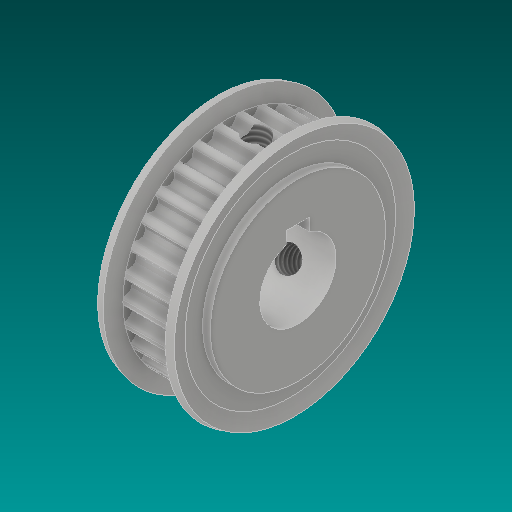
# Autodesk Inventor part: HTPA30S3M060-A-N10_b
Saved by Autodesk Inventor 2020 (Build 240168000, 168)
## iProperties
Created: 2022-11-15
Part Number: HTPA30S3M060-A-N10_b
Material: Generic
Catalog Web Link: www.cadenas.de
Description: HTPA__S3M060, HTPA__S3M100, HTPA__S3M150, HTPB__S3M060, HTPB__S3M100, HTPB__S3M150, HTPK__S3M060, HTPK__S3M100, HTPK__S3M150, HTPN__S3M060, HTPN__S3M100, HTPN__S3M150, HTPT__S3M060, HTPT__S3M100, HTPT__S3M150, HTPM__S3M060, HTPM__S3M100, HTPM__S3M150, HTPP__S3M060, HTPP__S3M100, HTPP__S3M150, HTPS__S3M060, HTPS__S3M100, KHTPA__S3M060, KHTPA__S3M100, KHTPA__S3M150, KHTPK__S3M060, KHTPK__S3M100, KHTPK__S3M150_body-High Torque Timing Pulleys S3M Type
Vendor: MISUMI
Document SubType Name: Modeling
Designer: psAdmin
Manufacturer: MISUMI
Mass: 5.31734 g
Surface Area: 36.0109 cm^2
Volume: 5.31734 cm^3
Density: 1 g/cm^3
Appearance: PSOLRGB-175-175-175
Category: PARTsolutions
Company: MISUMI
PSOL_IDENT_0: {$CADENAS_DATA/23d-libs/misumi/metric/51_timing_pulleys/htpk_s3m/htpa_s3m.prj},837 {VTYP=3D},{NB=HTP
PSOL_IDENT_1: A30S3M060-A-N10_b},{LINA=HTPA30S3M060-A-N10},{NN=HTPA__S3M060, HTPA__S3M100, HTPA__S3M150, HTPB__S3M
PSOL_IDENT_2: 060, HTPB__S3M100, HTPB__S3M150, HTPK__S3M060, HTPK__S3M100, HTPK__S3M150, HTPN__S3M060, HTPN__S3M10
PSOL_IDENT_3: 0, HTPN__S3M150, HTPT__S3M060, HTPT__S3M100, HTPT__S3M150, HTPM__S3M060, HTPM__S3M100, HTPM__S3M150,
PSOL_IDENT_4: HTPP__S3M060, HTPP__S3M100, HTPP__S3M150, HTPS__S3M060, HTPS__S3M100, KHTPA__S3M060, KHTPA__S3M100,
PSOL_IDENT_5: KHTPA__S3M150, KHTPK__S3M060, KHTPK__S3M100, KHTPK__S3M150_body},{DATE=28.10.2022 00:10:57},{GEOMDA
PSOL_IDENT_6: TE=11.11.2021 09:52:43},{VERSION=},{LINEID=160},{WBVAR=MATP,ST,TNW,PS,SBS,DD,Z,J,Q,R,S,T,ALT1,ALT2,M
PSOL_IDENT_7: ,QSC,QFC,QTC,ALT3,K,KSC,KFC,KTC,ALT4,ZM,ZSC,ZFC,ZTC,ALT5,ALT6,ALT7,FC,ALT8,SRG,ALT9,BTC,TL,ALT10,TPC
PSOL_IDENT_8: ,ALT11,BC,ALT12,SLH,ALT13,BN},{WBNUMERIC=DD,Z,J,Q,R,S,T,QSC,QFC,QTC,K,KSC,KFC,KTC,ZSC,ZFC,ZTC,FC,SRG
PSOL_IDENT_9: ,BTC,TL,BC,SLH,BN}  {NB=HTPA30S3M060-A-N10_b},{LINA=HTPA30S3M060-A-N10},{KT=DUMMY},{PN=HTPA30S3M060-
PSOL_IDENT_10: A-N10},{TYPE=HTPA},{MATP=A2017},{MATPALG='A2017','Aluminum Alloy 2000 series','S45C','1045 Carbon St
PSOL_IDENT_11: eel Equivalent','SUS304','304 Stainless Steel','A6000','6000 Series Aluminum Alloy'},{ST=CA},{STALG=
PSOL_IDENT_12: 'CA','Clear Anodize','BA','Black Anodize','HAT','Hard Clear Anodize','ENP','Electroless Nickel Plat
PSOL_IDENT_13: ing' },{NT=30},{TNW=S3M060},{TNWALG= 'S3M060','S3M100','S3M150'    },{BW=6},{PS=A},{PSALG='A','B'},{
PSOL_IDENT_14: SBS=N},{SBSALG= 'H','Round Hole','P','Round Hole + Tap','N','New JIS Keywayed Bore + Tap (Standard)'
PSOL_IDENT_15: ,'NK','New JIS Keywayed Bore + Tap (width 4.0mm, height 1.8mm)','C','Old JIS Keywayed Bore + Tap','V'
PSOL_IDENT_16: ,'Stepped Hole', 'Y','Both Ends Stepped Hole','WB', 'Double Stepped Hole' },{SHSA= 'H','Round Hole','
PSOL_IDENT_17: P','Round Hole + Tap','N','New JIS Keywayed Bore + Tap (Standard)','NK','New JIS Keywayed Bore + Tap
PSOL_IDENT_18: (width 4.0mm, height 1.8mm)','C','Old JIS Keywayed Bore + Tap','V','Stepped Hole', 'Y','Both Ends S
PSOL_IDENT_19: tepped Hole','WB', 'Double Stepped Hole' },{SHSB= 'H','Round Hole','P','Round Hole + Tap','N','New J
PSOL_IDENT_20: IS Keywayed Bore + Tap (Standard)','NK','New JIS Keywayed Bore + Tap (width 4.0mm, height 1.8mm)','C'
PSOL_IDENT_21: ,'Old JIS Keywayed Bore + Tap','V','Stepped Hole', 'F','Stepped Hole (Counterbore holes on the boss
PSOL_IDENT_22: side)'},{SHSK= '','' },{SBSPN=-N10},{DD=10.00},{DDALG=[8:8/1],[10:14/1]},{DDHA=[6:6/1],6.35,[7:12/1]
PSOL_IDENT_23: ,12.7,[13:19/1]},{DDHBK=0},{DDPA=[6:6/1],6.35,[7:12/1],12.7,[13:19/1]},{DDPBK=0},{DDNA=[8:8/1],[10:1
PSOL_IDENT_24: 4/1]},{DDNBK=0},{DDNK=10},{DDCA=[10:10/1],[12:12/1]},{DDCBK=0},{DDVA=[6:6/1],6.35,[7:12/1],12.7,[13:
PSOL_IDENT_25: 17/1]},{DDVF=[6:6/1],6.35,[7:12/1],12.7,[13:14/1]},{DDY=[6:17/1]},{DDWB=[6:15/1]},{Z=0},{ZALG=[0]},{
PSOL_IDENT_26: ZQRMIN=12},{ZAMAX=19},{ZBMAX=16},{DDZ=10},{J=0.0},{JALG=[0]},{JMAX=9},{JMIN=2},{JPN=},{QRMAX=19},{QR
PSOL_IDENT_27: MIN=12},{WBRMAX=-2.00},{WBQMIN=14},{Q=0},{QALG=[0]},{QPN=},{R=0},{RALG=[0]},{S=0.0},{SALG=[0]},{SPN=
PSOL_IDENT_28: },{SMAX=5},{T=0.0},{TALG=[0]},{TPN=},{TMAX=8},{A=7},{W=11},{L=0},{PD=28.65},{OD=27.89},{D=0},{DALG=2
PSOL_IDENT_29: 0},{DE=23},{F=32},{E=23},{BBK=3.000},{TTK=1.4},{TT=1},{ANG=120},{WL=11},{ALT1=},{ALT1ALG= '','w/o KC
PSOL_IDENT_30: 90 (Set Screw Angle)','KC90','with KC90 (Set Screw Angle)' },{ALT1PN=},{ALT2=},{ALT2ALG= '','Not app
PSOL_IDENT_31: licable' },{M=N/A},{MALG= 'N/A' },{MFTALG= 'N/A' },{MSALG= 'N/A' },{M3D=0.000},{KDML=0},{ML=0},{MUL=
PSOL_IDENT_32: 0},{PITCH=0},{QSC=0.0},{QSCALG=0},{QFC=0.0},{QFCALG=0},{QTC=0.0},{QTCALG=0},{QPCDMIN=0},{QPCDMINALG=
PSOL_IDENT_33: 0},{QPCDMAX=19},{ALT2PN=},{ALT3=},{ALT3ALG= '','Not applicable' },{K=0.0},{KALG=0},{KMIN=4},{KFTMAX=
PSOL_IDENT_34: 0.0},{KSMAX=0.0},{KSC=0.0},{KSCALG=0},{KFC=0.0},{KFCALG=0},{KTC=0.0},{KTCALG=0},{KPCDMIN=14},{KPCDMI
PSOL_IDENT_35: NALG=14},{KPCDMAX=19},{KSCMIN=14.0},{KSCMINALG=14},{ALT3PN=},{ALT4=},{ALT4ALG= '','Not applicable' }
PSOL_IDENT_36: ,{ALT4MIN=20.5},{ALT4MAX=12.5},{ZM=N/A},{ZMALG= 'N/A' },{ZMSALG= 'N/A' },{ZMFTALG= 'N/A' },{ZMDD1=0.
PSOL_IDENT_37: 0},{ZMDD2=0.0},{ZMHH=0.0},{ZSC=0.0},{ZSCALG=[0]},{ZFC=0.0},{ZFCALG=[0]},{ZTC=0.0},{ZTCALG=[0]},{ZPCD
PSOL_IDENT_38: MIN=0},{ZPCDMINALG=0},{ZPCDMAX=19},{ALT4PN=},{ALT5=},{ALT5ALG= '','Flange Attached','NFC','with NFC
PSOL_IDENT_39: (Flange not Attached)' },{ALT5PN=},{ALT6=},{ALT6ALG= '','w/o Flange Attached on One Side Only','RFC'
PSOL_IDENT_40: ,'with RFC (Flange Attached on The Boss Side Only)','LFC','with LFC (Flange Attached on The Opposite
PSOL_IDENT_41: Side Only)' },{ALT6PN=},{ALT7=},{ALT7ALG= '','w/o FC (Flange Cut)','FC','with FC (Flange Cut)' },{F
PSOL_IDENT_42: C=0.0},{FCALG=0},{FCMIN=29.0},{FCMAX=30.0},{ALT7PN=},{ALT8=},{ALT8ALG= '','Not applicable' },{ALT8AL
PSOL_IDENT_43: GALG=19},{ALT8DD2=0},{ALT8MM=0},{ALT8NN=0},{QC=0},{KC=0},{ZC=0},{SRG=0.0},{SRGALG=[0]},{SRGMAX1=0},{
PSOL_IDENT_44: SRGMAX=0},{DD2=0.0},{MM=0.00},{NN=0.00},{ALT8PN=},{ALT9ALG= '','Not applicable' },{ALT9=},{BTC9=11},
PSOL_IDENT_45: {TL9=1},{BTC=0},{BTCALG=[0]},{TL=0.0},{TLALG=0},{TLMIN=1.0},{TLMAX=-11.5},{BTCL=0},{BTCD=0},{BTCDALG=
PSOL_IDENT_46: 20.000},{ALT9PN=},{WLBCTL=11},{ALT10=},{ALT10ALG= '','w/o TPC (Tapped Hole Dimension)','TPC','with T
PSOL_IDENT_47: PC (Tapped Hole Dimension)' },{TPC=N/A},{TPCALG= 'N/A' },{TPCM=4},{ALT10PN=},{ALT11=},{ALT11ALG= '','
PSOL_IDENT_48: Not applicable' },{BC=0.0},{BCALG=0},{BCMIN=7},{BCMAX=-11.5},{BCPLANE=5.5},{M1WBC=5.5},{ALT11PN=},{A
PSOL_IDENT_49: LT12=},{ALT12ALG= '','w/o SLH (Set Screw Length)','SLH','with SLH (Set Screw Length)' },{SLH=0},{SLH
PSOL_IDENT_50: ALG=[0]},{ALT12PN=},{AC=M4x3},{M1=4},{M1L=3},{TAP=0.000},{KYY=5},{KTT=8.945},{PLANE=11},{CD=0},{ALT1
PSOL_IDENT_51: 3=},{ALT13ALG= '', 'Not applicable' },{BN=0.0},{BNALG=0},{BNMIN=-10.5},{BNMAX=-1.0},{ALT13PN=}
NB: HTPA30S3M060-A-N10_b
NN: 0
NT: 30
NBSYN: $PN._b
LINA: HTPA30S3M060-A-N10
CATALOG: Misumi
PN: HTPA30S3M060-A-N10
MATP: Aluminum Alloy 2000 series
ST: Clear Anodize
TNW: S3M060
BW: 6
PS: A
SBS: New JIS Keywayed Bore + Tap (Standard)
DD: 10
Z: 0
J: 0
Q: 0
R: 0
S: 0
T: 0
A: 7
W: 11
L: 0
PD: 28.65
OD: 27.89
D: 0
F: 32
E: 23
TT: 1
ALT1: w/o KC90 (Set Screw Angle)
ALT2: Not applicable
M: N/A
QSC: 0
QFC: 0
QTC: 0
ALT3: Not applicable
K: 0
KSC: 0
KFC: 0
KTC: 0
ALT4: Not applicable
ZM: N/A
ZMDD1: 0
ZMDD2: 0
ZMHH: 0
ZSC: 0
ZFC: 0
ZTC: 0
ALT5: Flange Attached
ALT6: w/o Flange Attached on One Side Only
ALT7: w/o FC (Flange Cut)
FC: 0
ALT8: Not applicable
SRG: 0
DD2: 0
MM: 0
ALT9: Not applicable
BTC: 0
TL: 0
BTCL: 0
BTCD: 0
ALT10: w/o TPC (Tapped Hole Dimension)
TPC: N/A
ALT11: Not applicable
BC: 0
ALT12: w/o SLH (Set Screw Length)
SLH: 0
AC: M4x3
ALT13: Not applicable
BN: 0
SUPPLIER: MISUMI
ARTICLENO: HTPA30S3M060-A-N10_b
BOMINFO: HTPA30S3M060-A-N10
CREATOR: CADENAS GmbH
d18: 0.000 mm
Title: HTPA30S3M060-A-N10
Author: Cadenas PARTsolutions
Comments: High Torque Timing Pulleys S3M Type
Autodesk Inventor part; units mm, degrees
ref_plane "YZ Plane" through (0, 0, 0) normal (1, 0, 0) x (0, 1, 0)
ref_plane "XZ Plane" through (0, 0, 0) normal (0, 1, 0) x (-1, 0, 0)
ref_plane "XY Plane" through (0, 0, 0) normal (0, 0, 1) x (1, 0, 0)
sketch "_____1" plane through (0, 0, 0) normal (0, 0, 1) x (1, 0, 0)
  line L0 (11, 0) -> (0, 0)
  line L1 (0, 0) -> (0, 11.5)
  line L2 (0, 11.5) -> (1, 11.5)
  line L3 (1, 11.5) -> (1, 13.8133)
  line L4 (1, 13.8133) -> (0.4834, 15.7412)
  line L5 (0.4834, 15.7412) -> (1.4494, 16)
  line L6 (1.4494, 16) -> (2, 13.945)
  line L7 (2, 13.945) -> (9, 13.945)
  line L8 (9, 13.945) -> (9.5506, 16)
  line L9 (9.5506, 16) -> (10.5166, 15.7412)
  line L10 (10.5166, 15.7412) -> (10, 13.8133)
  line L11 (10, 13.8133) -> (10, 11.5)
  line L12 (10, 11.5) -> (11, 11.5)
  line L13 (11, 11.5) -> (11, 0)
  line L14 (11, 0) -> (0, 0)
  constraints: 30 end point
revolve "Revolution1" add sketch "_____1" angle 360 about axis through (11, 0, 0) along (1, 0, 0)
sketch "Sketch2" plane through (11, 0, 0) normal (1, 0, 0) x (0, 0, -1)
  point P0 (0, 0)
hole "Hole1" at (11, 0, 0) direction (-1, 0, 0) diameter 10 depth 11
sketch "_____6" plane through (2, 0, 0) normal (1, 0, 0) x (0, 0, -1)
  circle A0 centre (0, 0) radius 18.945
  arc A1 (-13.9426, 0.2589) -> (-13.9426, -0.2589) centre (0, 0) ccw
  arc A2 (-13.9426, -0.2589) -> (-13.7184, -0.5281) centre (-13.6626, -0.2537) ccw
  arc A3 (-12.8452, -0.948) -> (-13.7184, -0.5281) centre (-14.1116, -2.4636) ccw
  arc A4 (-12.7919, -1.0508) -> (-12.8452, -0.948) centre (-12.9414, -1.0631) ccw
  arc A5 (-12.7919, -1.0508) -> (-12.7309, -1.6318) centre (0, 0) ccw
  arc A6 (-12.7616, -1.7434) -> (-12.7309, -1.6318) centre (-12.8796, -1.6508) ccw
  arc A7 (-13.5284, -2.3357) -> (-12.7616, -1.7434) centre (-14.3154, -0.5242) ccw
  arc A8 (-13.5284, -2.3357) -> (-13.6917, -2.6456) centre (-13.4168, -2.5925) ccw
  arc A9 (-13.6917, -2.6456) -> (-13.5841, -3.1521) centre (0, 0) ccw
  arc A10 (-13.5841, -3.1521) -> (-13.3088, -3.3688) centre (-13.3113, -3.0888) ccw
  arc A11 (-12.3674, -3.5979) -> (-13.3088, -3.3688) centre (-13.291, -5.3437) ccw
  arc A12 (-12.2939, -3.6874) -> (-12.3674, -3.5979) centre (-12.4376, -3.7305) ccw
  arc A13 (-12.2939, -3.6874) -> (-12.1134, -4.243) centre (0, 0) ccw
  arc A14 (-12.1203, -4.3586) -> (-12.1134, -4.243) centre (-12.255, -4.2926) ccw
  arc A15 (-12.7472, -5.0973) -> (-12.1203, -4.3586) centre (-13.8936, -3.4891) ccw
  arc A16 (-12.7472, -5.0973) -> (-12.8425, -5.4345) centre (-12.5846, -5.3253) ccw
  arc A17 (-12.8425, -5.4345) -> (-12.6319, -5.9075) centre (0, 0) ccw
  arc A18 (-12.6319, -5.9075) -> (-12.3176, -6.0622) centre (-12.3783, -5.7889) ccw
  arc A19 (-11.3491, -6.0906) -> (-12.3176, -6.0622) centre (-11.8895, -7.9903) ccw
  arc A20 (-11.2586, -6.1629) -> (-11.3491, -6.0906) centre (-11.3902, -6.2349) ccw
  arc A21 (-11.2586, -6.1629) -> (-10.9665, -6.6688) centre (0, 0) ccw
  arc A22 (-10.9492, -6.7833) -> (-10.9665, -6.6688) centre (-11.0947, -6.7467) ccw
  arc A23 (-11.4088, -7.6362) -> (-10.9492, -6.7833) centre (-12.8645, -6.3015) ccw
  arc A24 (-11.4088, -7.6362) -> (-11.432, -7.9858) centre (-11.2024, -7.8255) ccw
  arc A25 (-11.432, -7.9858) -> (-11.1276, -8.4047) centre (0, 0) ccw
  arc A26 (-11.1276, -8.4047) -> (-10.788, -8.4907) centre (-10.9042, -8.2359) ccw
  arc A27 (-9.8348, -8.3172) -> (-10.788, -8.4907) centre (-9.9685, -10.2876) ccw
  arc A28 (-9.7312, -8.369) -> (-9.8348, -8.3172) centre (-9.845, -8.4668) ccw
  arc A29 (-9.7312, -8.369) -> (-9.3404, -8.8031) centre (0, 0) ccw
  arc A30 (-9.2996, -8.9116) -> (-9.3404, -8.8031) centre (-9.4495, -8.906) ccw
  arc A31 (-9.5718, -9.8414) -> (-9.2996, -8.9116) centre (-11.2733, -8.8385) ccw
  arc A32 (-9.5718, -9.8414) -> (-9.5218, -10.1881) centre (-9.3306, -9.9836) ccw
  arc A33 (-9.5218, -10.1881) -> (-9.137, -10.5346) centre (0, 0) ccw
  arc A34 (-9.137, -10.5346) -> (-8.7869, -10.5481) centre (-8.9536, -10.3231) ccw
  arc A35 (-7.8907, -10.1802) -> (-8.7869, -10.5481) centre (-7.6117, -12.1354) ccw
  arc A36 (-7.7786, -10.2094) -> (-7.8907, -10.1802) centre (-7.8695, -10.3287) ccw
  arc A37 (-7.7786, -10.2094) -> (-7.306, -10.5527) centre (0, 0) ccw
  arc A38 (-7.2436, -10.6503) -> (-7.306, -10.5527) centre (-7.3914, -10.6761) ccw
  arc A39 (-7.3165, -11.6164) -> (-7.2436, -10.6503) centre (-9.1893, -10.9892) ccw
  arc A40 (-7.3165, -11.6164) -> (-7.1955, -11.9452) centre (-7.051, -11.7053) ccw
  arc A41 (-7.1955, -11.9452) -> (-6.7471, -12.2041) centre (0, 0) ccw
  arc A42 (-6.7471, -12.2041) -> (-6.4019, -12.1445) centre (-6.6116, -11.959) ccw
  arc A43 (-5.6017, -11.5983) -> (-6.4019, -12.1445) centre (-4.9223, -13.4528) ccw
  arc A44 (-5.4859, -11.6035) -> (-5.6017, -11.5983) centre (-5.5501, -11.7391) ccw
  arc A45 (-5.4859, -11.6035) -> (-4.9523, -11.8411) centre (0, 0) ccw
  arc A46 (-4.871, -11.9236) -> (-4.9523, -11.8411) centre (-5.0102, -11.9795) ccw
  arc A47 (-4.7415, -12.8838) -> (-4.871, -11.9236) centre (-6.7037, -12.6596) ccw
  arc A48 (-4.7415, -12.8838) -> (-4.5547, -13.1802) centre (-4.4633, -12.9156) ccw
  arc A49 (-4.5547, -13.1802) -> (-4.0623, -13.3402) centre (0, 0) ccw
  arc A50 (-4.0623, -13.3402) -> (-3.737, -13.2102) centre (-3.9807, -13.0723) ccw
  arc A51 (-3.0678, -12.5095) -> (-3.737, -13.2102) centre (-2.0177, -14.1822) ccw
  arc A52 (-2.9536, -12.4905) -> (-3.0678, -12.5095) centre (-2.9881, -12.6365) ccw
  arc A53 (-2.9536, -12.4905) -> (-2.3822, -12.612) centre (0, 0) ccw
  arc A54 (-2.2855, -12.6758) -> (-2.3822, -12.612) centre (-2.41, -12.7594) ccw
  arc A55 (-1.9592, -13.588) -> (-2.2855, -12.6758) centre (-3.9251, -13.7768) ccw
  arc A56 (-1.9592, -13.588) -> (-1.7149, -13.8392) centre (-1.6804, -13.5613) ccw
  arc A57 (-1.7149, -13.8392) -> (-1.1999, -13.8933) centre (0, 0) ccw
  arc A58 (-1.1999, -13.8933) -> (-0.9088, -13.6984) centre (-1.1758, -13.6143) ccw
  arc A59 (-0.3999, -12.874) -> (-0.9088, -13.6984) centre (0.975, -14.2918) ccw
  arc A60 (-0.2921, -12.8317) -> (-0.3999, -12.874) centre (-0.2955, -12.9816) ccw
  arc A61 (-0.2921, -12.8317) -> (0.2921, -12.8317) centre (0, 0) ccw
  arc A62 (0.3999, -12.874) -> (0.2921, -12.8317) centre (0.2955, -12.9816) ccw
  arc A63 (0.9088, -13.6984) -> (0.3999, -12.874) centre (-0.975, -14.2918) ccw
  arc A64 (0.9088, -13.6984) -> (1.1999, -13.8933) centre (1.1758, -13.6143) ccw
  arc A65 (1.1999, -13.8933) -> (1.7149, -13.8392) centre (0, 0) ccw
  arc A66 (1.7149, -13.8392) -> (1.9592, -13.588) centre (1.6804, -13.5613) ccw
  arc A67 (2.2855, -12.6758) -> (1.9592, -13.588) centre (3.9251, -13.7768) ccw
  arc A68 (2.3822, -12.612) -> (2.2855, -12.6758) centre (2.41, -12.7594) ccw
  arc A69 (2.3822, -12.612) -> (2.9536, -12.4905) centre (0, 0) ccw
  arc A70 (3.0678, -12.5095) -> (2.9536, -12.4905) centre (2.9881, -12.6365) ccw
  arc A71 (3.737, -13.2102) -> (3.0678, -12.5095) centre (2.0177, -14.1822) ccw
  arc A72 (3.737, -13.2102) -> (4.0623, -13.3402) centre (3.9807, -13.0723) ccw
  arc A73 (4.0623, -13.3402) -> (4.5547, -13.1802) centre (0, 0) ccw
  arc A74 (4.5547, -13.1802) -> (4.7415, -12.8838) centre (4.4633, -12.9156) ccw
  arc A75 (4.871, -11.9236) -> (4.7415, -12.8838) centre (6.7037, -12.6596) ccw
  arc A76 (4.9523, -11.8411) -> (4.871, -11.9236) centre (5.0102, -11.9795) ccw
  arc A77 (4.9523, -11.8411) -> (5.4859, -11.6035) centre (0, 0) ccw
  arc A78 (5.6017, -11.5983) -> (5.4859, -11.6035) centre (5.5501, -11.7391) ccw
  arc A79 (6.4019, -12.1445) -> (5.6017, -11.5983) centre (4.9223, -13.4528) ccw
  arc A80 (6.4019, -12.1445) -> (6.7471, -12.2041) centre (6.6116, -11.959) ccw
  arc A81 (6.7471, -12.2041) -> (7.1955, -11.9452) centre (0, 0) ccw
  arc A82 (7.1955, -11.9452) -> (7.3165, -11.6164) centre (7.051, -11.7053) ccw
  arc A83 (7.2436, -10.6503) -> (7.3165, -11.6164) centre (9.1893, -10.9892) ccw
  arc A84 (7.306, -10.5527) -> (7.2436, -10.6503) centre (7.3914, -10.6761) ccw
  arc A85 (7.306, -10.5527) -> (7.7786, -10.2094) centre (0, 0) ccw
  arc A86 (7.8907, -10.1802) -> (7.7786, -10.2094) centre (7.8695, -10.3287) ccw
  arc A87 (8.7869, -10.5481) -> (7.8907, -10.1802) centre (7.6117, -12.1354) ccw
  arc A88 (8.7869, -10.5481) -> (9.137, -10.5346) centre (8.9536, -10.3231) ccw
  arc A89 (9.137, -10.5346) -> (9.5218, -10.1881) centre (0, 0) ccw
  arc A90 (9.5218, -10.1881) -> (9.5718, -9.8414) centre (9.3306, -9.9836) ccw
  arc A91 (9.2996, -8.9116) -> (9.5718, -9.8414) centre (11.2733, -8.8385) ccw
  arc A92 (9.3404, -8.8031) -> (9.2996, -8.9116) centre (9.4495, -8.906) ccw
  arc A93 (9.3404, -8.8031) -> (9.7312, -8.369) centre (0, 0) ccw
  arc A94 (9.8348, -8.3172) -> (9.7312, -8.369) centre (9.845, -8.4668) ccw
  arc A95 (10.788, -8.4907) -> (9.8348, -8.3172) centre (9.9685, -10.2876) ccw
  arc A96 (10.788, -8.4907) -> (11.1276, -8.4047) centre (10.9042, -8.2359) ccw
  arc A97 (11.1276, -8.4047) -> (11.432, -7.9858) centre (0, 0) ccw
  arc A98 (11.432, -7.9858) -> (11.4088, -7.6362) centre (11.2024, -7.8255) ccw
  arc A99 (10.9492, -6.7833) -> (11.4088, -7.6362) centre (12.8645, -6.3015) ccw
  arc A100 (10.9665, -6.6688) -> (10.9492, -6.7833) centre (11.0947, -6.7467) ccw
  arc A101 (10.9665, -6.6688) -> (11.2586, -6.1629) centre (0, 0) ccw
  arc A102 (11.3491, -6.0906) -> (11.2586, -6.1629) centre (11.3902, -6.2349) ccw
  arc A103 (12.3176, -6.0622) -> (11.3491, -6.0906) centre (11.8895, -7.9903) ccw
  arc A104 (12.3176, -6.0622) -> (12.6319, -5.9075) centre (12.3783, -5.7889) ccw
  arc A105 (12.6319, -5.9075) -> (12.8425, -5.4345) centre (0, 0) ccw
  arc A106 (12.8425, -5.4345) -> (12.7472, -5.0973) centre (12.5846, -5.3253) ccw
  arc A107 (12.1203, -4.3586) -> (12.7472, -5.0973) centre (13.8936, -3.4891) ccw
  arc A108 (12.1134, -4.243) -> (12.1203, -4.3586) centre (12.255, -4.2926) ccw
  arc A109 (12.1134, -4.243) -> (12.2939, -3.6874) centre (0, 0) ccw
  arc A110 (12.3674, -3.5979) -> (12.2939, -3.6874) centre (12.4376, -3.7305) ccw
  arc A111 (13.3088, -3.3688) -> (12.3674, -3.5979) centre (13.291, -5.3437) ccw
  arc A112 (13.3088, -3.3688) -> (13.5841, -3.1521) centre (13.3113, -3.0888) ccw
  arc A113 (13.5841, -3.1521) -> (13.6917, -2.6456) centre (0, 0) ccw
  arc A114 (13.6917, -2.6456) -> (13.5284, -2.3357) centre (13.4168, -2.5925) ccw
  arc A115 (12.7616, -1.7434) -> (13.5284, -2.3357) centre (14.3154, -0.5242) ccw
  arc A116 (12.7309, -1.6318) -> (12.7616, -1.7434) centre (12.8796, -1.6508) ccw
  arc A117 (12.7309, -1.6318) -> (12.7919, -1.0508) centre (0, 0) ccw
  arc A118 (12.8452, -0.948) -> (12.7919, -1.0508) centre (12.9414, -1.0631) ccw
  arc A119 (13.7184, -0.5281) -> (12.8452, -0.948) centre (14.1116, -2.4636) ccw
  arc A120 (13.7184, -0.5281) -> (13.9426, -0.2589) centre (13.6626, -0.2537) ccw
  arc A121 (13.9426, -0.2589) -> (13.9426, 0.2589) centre (0, 0) ccw
  arc A122 (13.9426, 0.2589) -> (13.7184, 0.5281) centre (13.6626, 0.2537) ccw
  arc A123 (12.8452, 0.948) -> (13.7184, 0.5281) centre (14.1116, 2.4636) ccw
  arc A124 (12.7919, 1.0508) -> (12.8452, 0.948) centre (12.9414, 1.0631) ccw
  arc A125 (12.7919, 1.0508) -> (12.7309, 1.6318) centre (0, 0) ccw
  arc A126 (12.7616, 1.7434) -> (12.7309, 1.6318) centre (12.8796, 1.6508) ccw
  arc A127 (13.5284, 2.3357) -> (12.7616, 1.7434) centre (14.3154, 0.5242) ccw
  arc A128 (13.5284, 2.3357) -> (13.6917, 2.6456) centre (13.4168, 2.5925) ccw
  arc A129 (13.6917, 2.6456) -> (13.5841, 3.1521) centre (0, 0) ccw
  arc A130 (13.5841, 3.1521) -> (13.3088, 3.3688) centre (13.3113, 3.0888) ccw
  arc A131 (12.3674, 3.5979) -> (13.3088, 3.3688) centre (13.291, 5.3437) ccw
  arc A132 (12.2939, 3.6874) -> (12.3674, 3.5979) centre (12.4376, 3.7305) ccw
  arc A133 (12.2939, 3.6874) -> (12.1134, 4.243) centre (0, 0) ccw
  arc A134 (12.1203, 4.3586) -> (12.1134, 4.243) centre (12.255, 4.2926) ccw
  arc A135 (12.7472, 5.0973) -> (12.1203, 4.3586) centre (13.8936, 3.4891) ccw
  arc A136 (12.7472, 5.0973) -> (12.8425, 5.4345) centre (12.5846, 5.3253) ccw
  arc A137 (12.8425, 5.4345) -> (12.6319, 5.9075) centre (0, 0) ccw
  arc A138 (12.6319, 5.9075) -> (12.3176, 6.0622) centre (12.3783, 5.7889) ccw
  arc A139 (11.3491, 6.0906) -> (12.3176, 6.0622) centre (11.8895, 7.9903) ccw
  arc A140 (11.2586, 6.1629) -> (11.3491, 6.0906) centre (11.3902, 6.2349) ccw
  arc A141 (11.2586, 6.1629) -> (10.9665, 6.6688) centre (0, 0) ccw
  arc A142 (10.9492, 6.7833) -> (10.9665, 6.6688) centre (11.0947, 6.7467) ccw
  arc A143 (11.4088, 7.6362) -> (10.9492, 6.7833) centre (12.8645, 6.3015) ccw
  arc A144 (11.4088, 7.6362) -> (11.432, 7.9858) centre (11.2024, 7.8255) ccw
  arc A145 (11.432, 7.9858) -> (11.1276, 8.4047) centre (0, 0) ccw
  arc A146 (11.1276, 8.4047) -> (10.788, 8.4907) centre (10.9042, 8.2359) ccw
  arc A147 (9.8348, 8.3172) -> (10.788, 8.4907) centre (9.9685, 10.2876) ccw
  arc A148 (9.7312, 8.369) -> (9.8348, 8.3172) centre (9.845, 8.4668) ccw
  arc A149 (9.7312, 8.369) -> (9.3404, 8.8031) centre (0, 0) ccw
  arc A150 (9.2996, 8.9116) -> (9.3404, 8.8031) centre (9.4495, 8.906) ccw
  arc A151 (9.5718, 9.8414) -> (9.2996, 8.9116) centre (11.2733, 8.8385) ccw
  arc A152 (9.5718, 9.8414) -> (9.5218, 10.1881) centre (9.3306, 9.9836) ccw
  arc A153 (9.5218, 10.1881) -> (9.137, 10.5346) centre (0, 0) ccw
  arc A154 (9.137, 10.5346) -> (8.7869, 10.5481) centre (8.9536, 10.3231) ccw
  arc A155 (7.8907, 10.1802) -> (8.7869, 10.5481) centre (7.6117, 12.1354) ccw
  arc A156 (7.7786, 10.2094) -> (7.8907, 10.1802) centre (7.8695, 10.3287) ccw
  arc A157 (7.7786, 10.2094) -> (7.306, 10.5527) centre (0, 0) ccw
  arc A158 (7.2436, 10.6503) -> (7.306, 10.5527) centre (7.3914, 10.6761) ccw
  arc A159 (7.3165, 11.6164) -> (7.2436, 10.6503) centre (9.1893, 10.9892) ccw
  arc A160 (7.3165, 11.6164) -> (7.1955, 11.9452) centre (7.051, 11.7053) ccw
  arc A161 (7.1955, 11.9452) -> (6.7471, 12.2041) centre (0, 0) ccw
  arc A162 (6.7471, 12.2041) -> (6.4019, 12.1445) centre (6.6116, 11.959) ccw
  arc A163 (5.6017, 11.5983) -> (6.4019, 12.1445) centre (4.9223, 13.4528) ccw
  arc A164 (5.4859, 11.6035) -> (5.6017, 11.5983) centre (5.5501, 11.7391) ccw
  arc A165 (5.4859, 11.6035) -> (4.9523, 11.8411) centre (0, 0) ccw
  arc A166 (4.871, 11.9236) -> (4.9523, 11.8411) centre (5.0102, 11.9795) ccw
  arc A167 (4.7415, 12.8838) -> (4.871, 11.9236) centre (6.7037, 12.6596) ccw
  arc A168 (4.7415, 12.8838) -> (4.5547, 13.1802) centre (4.4633, 12.9156) ccw
  arc A169 (4.5547, 13.1802) -> (4.0623, 13.3402) centre (0, 0) ccw
  arc A170 (4.0623, 13.3402) -> (3.737, 13.2102) centre (3.9807, 13.0723) ccw
  arc A171 (3.0678, 12.5095) -> (3.737, 13.2102) centre (2.0177, 14.1822) ccw
  arc A172 (2.9536, 12.4905) -> (3.0678, 12.5095) centre (2.9881, 12.6365) ccw
  arc A173 (2.9536, 12.4905) -> (2.3822, 12.612) centre (0, 0) ccw
  arc A174 (2.2855, 12.6758) -> (2.3822, 12.612) centre (2.41, 12.7594) ccw
  arc A175 (1.9592, 13.588) -> (2.2855, 12.6758) centre (3.9251, 13.7768) ccw
  arc A176 (1.9592, 13.588) -> (1.7149, 13.8392) centre (1.6804, 13.5613) ccw
  arc A177 (1.7149, 13.8392) -> (1.1999, 13.8933) centre (0, 0) ccw
  arc A178 (1.1999, 13.8933) -> (0.9088, 13.6984) centre (1.1758, 13.6143) ccw
  arc A179 (0.3999, 12.874) -> (0.9088, 13.6984) centre (-0.975, 14.2918) ccw
  arc A180 (0.2921, 12.8317) -> (0.3999, 12.874) centre (0.2955, 12.9816) ccw
  arc A181 (0.2921, 12.8317) -> (-0.2921, 12.8317) centre (0, 0) ccw
  arc A182 (-0.3999, 12.874) -> (-0.2921, 12.8317) centre (-0.2955, 12.9816) ccw
  arc A183 (-0.9088, 13.6984) -> (-0.3999, 12.874) centre (0.975, 14.2918) ccw
  arc A184 (-0.9088, 13.6984) -> (-1.1999, 13.8933) centre (-1.1758, 13.6143) ccw
  arc A185 (-1.1999, 13.8933) -> (-1.7149, 13.8392) centre (0, 0) ccw
  arc A186 (-1.7149, 13.8392) -> (-1.9592, 13.588) centre (-1.6804, 13.5613) ccw
  arc A187 (-2.2855, 12.6758) -> (-1.9592, 13.588) centre (-3.9251, 13.7768) ccw
  arc A188 (-2.3822, 12.612) -> (-2.2855, 12.6758) centre (-2.41, 12.7594) ccw
  arc A189 (-2.3822, 12.612) -> (-2.9536, 12.4905) centre (0, 0) ccw
  arc A190 (-3.0678, 12.5095) -> (-2.9536, 12.4905) centre (-2.9881, 12.6365) ccw
  arc A191 (-3.737, 13.2102) -> (-3.0678, 12.5095) centre (-2.0177, 14.1822) ccw
  arc A192 (-3.737, 13.2102) -> (-4.0623, 13.3402) centre (-3.9807, 13.0723) ccw
  arc A193 (-4.0623, 13.3402) -> (-4.5547, 13.1802) centre (0, 0) ccw
  arc A194 (-4.5547, 13.1802) -> (-4.7415, 12.8838) centre (-4.4633, 12.9156) ccw
  arc A195 (-4.871, 11.9236) -> (-4.7415, 12.8838) centre (-6.7037, 12.6596) ccw
  arc A196 (-4.9523, 11.8411) -> (-4.871, 11.9236) centre (-5.0102, 11.9795) ccw
  arc A197 (-4.9523, 11.8411) -> (-5.4859, 11.6035) centre (0, 0) ccw
  arc A198 (-5.6017, 11.5983) -> (-5.4859, 11.6035) centre (-5.5501, 11.7391) ccw
  arc A199 (-6.4019, 12.1445) -> (-5.6017, 11.5983) centre (-4.9223, 13.4528) ccw
  arc A200 (-6.4019, 12.1445) -> (-6.7471, 12.2041) centre (-6.6116, 11.959) ccw
  arc A201 (-6.7471, 12.2041) -> (-7.1955, 11.9452) centre (0, 0) ccw
  arc A202 (-7.1955, 11.9452) -> (-7.3165, 11.6164) centre (-7.051, 11.7053) ccw
  arc A203 (-7.2436, 10.6503) -> (-7.3165, 11.6164) centre (-9.1893, 10.9892) ccw
  arc A204 (-7.306, 10.5527) -> (-7.2436, 10.6503) centre (-7.3914, 10.6761) ccw
  arc A205 (-7.306, 10.5527) -> (-7.7786, 10.2094) centre (0, 0) ccw
  arc A206 (-7.8907, 10.1802) -> (-7.7786, 10.2094) centre (-7.8695, 10.3287) ccw
  arc A207 (-8.7869, 10.5481) -> (-7.8907, 10.1802) centre (-7.6117, 12.1354) ccw
  arc A208 (-8.7869, 10.5481) -> (-9.137, 10.5346) centre (-8.9536, 10.3231) ccw
  arc A209 (-9.137, 10.5346) -> (-9.5218, 10.1881) centre (0, 0) ccw
  arc A210 (-9.5218, 10.1881) -> (-9.5718, 9.8414) centre (-9.3306, 9.9836) ccw
  arc A211 (-9.2996, 8.9116) -> (-9.5718, 9.8414) centre (-11.2733, 8.8385) ccw
  arc A212 (-9.3404, 8.8031) -> (-9.2996, 8.9116) centre (-9.4495, 8.906) ccw
  arc A213 (-9.3404, 8.8031) -> (-9.7312, 8.369) centre (0, 0) ccw
  arc A214 (-9.8348, 8.3172) -> (-9.7312, 8.369) centre (-9.845, 8.4668) ccw
  arc A215 (-10.788, 8.4907) -> (-9.8348, 8.3172) centre (-9.9685, 10.2876) ccw
  arc A216 (-10.788, 8.4907) -> (-11.1276, 8.4047) centre (-10.9042, 8.2359) ccw
  arc A217 (-11.1276, 8.4047) -> (-11.432, 7.9858) centre (0, 0) ccw
  arc A218 (-11.432, 7.9858) -> (-11.4088, 7.6362) centre (-11.2024, 7.8255) ccw
  arc A219 (-10.9492, 6.7833) -> (-11.4088, 7.6362) centre (-12.8645, 6.3015) ccw
  arc A220 (-10.9665, 6.6688) -> (-10.9492, 6.7833) centre (-11.0947, 6.7467) ccw
  arc A221 (-10.9665, 6.6688) -> (-11.2586, 6.1629) centre (0, 0) ccw
  arc A222 (-11.3491, 6.0906) -> (-11.2586, 6.1629) centre (-11.3902, 6.2349) ccw
  arc A223 (-12.3176, 6.0622) -> (-11.3491, 6.0906) centre (-11.8895, 7.9903) ccw
  arc A224 (-12.3176, 6.0622) -> (-12.6319, 5.9075) centre (-12.3783, 5.7889) ccw
  arc A225 (-12.6319, 5.9075) -> (-12.8425, 5.4345) centre (0, 0) ccw
  arc A226 (-12.8425, 5.4345) -> (-12.7472, 5.0973) centre (-12.5846, 5.3253) ccw
  arc A227 (-12.1203, 4.3586) -> (-12.7472, 5.0973) centre (-13.8936, 3.4891) ccw
  arc A228 (-12.1134, 4.243) -> (-12.1203, 4.3586) centre (-12.255, 4.2926) ccw
  arc A229 (-12.1134, 4.243) -> (-12.2939, 3.6874) centre (0, 0) ccw
  arc A230 (-12.3674, 3.5979) -> (-12.2939, 3.6874) centre (-12.4376, 3.7305) ccw
  arc A231 (-13.3088, 3.3688) -> (-12.3674, 3.5979) centre (-13.291, 5.3437) ccw
  arc A232 (-13.3088, 3.3688) -> (-13.5841, 3.1521) centre (-13.3113, 3.0888) ccw
  arc A233 (-13.5841, 3.1521) -> (-13.6917, 2.6456) centre (0, 0) ccw
  arc A234 (-13.6917, 2.6456) -> (-13.5284, 2.3357) centre (-13.4168, 2.5925) ccw
  arc A235 (-12.7616, 1.7434) -> (-13.5284, 2.3357) centre (-14.3154, 0.5242) ccw
  arc A236 (-12.7309, 1.6318) -> (-12.7616, 1.7434) centre (-12.8796, 1.6508) ccw
  arc A237 (-12.7309, 1.6318) -> (-12.7919, 1.0508) centre (0, 0) ccw
  arc A238 (-12.8452, 0.948) -> (-12.7919, 1.0508) centre (-12.9414, 1.0631) ccw
  arc A239 (-13.7184, 0.5281) -> (-12.8452, 0.948) centre (-14.1116, 2.4636) ccw
  arc A240 (-13.7184, 0.5281) -> (-13.9426, 0.2589) centre (-13.6626, 0.2537) ccw
  constraints: 480 point on circle, 241 centre point
extrude "Extrusion1" cut sketch "_____6" along normal blind 7
sketch "_____10" plane through (0, 0, 0) normal (1, 0, 0) x (0, 0, -1)
  line L0 (-1.5, 6.4) -> (-1.5, 0)
  line L1 (-1.5, 0) -> (1.5, 0)
  line L2 (1.5, 0) -> (1.5, 6.4)
  line L3 (1.5, 6.4) -> (-1.5, 6.4)
  constraints: 8 end point
extrude "Extrusion2" cut sketch "_____10" along normal blind 11
sketch "_____18" plane through (5.5, 0, 0) normal (1, 0, 0) x (0, 0, -1)
  line L0 (0, 0) -> (0, 13.945)
  line L1 (0, 13.945) -> (1.621, 13.945)
  line L2 (1.621, 13.945) -> (1.621, 0)
  line L3 (1.621, 0) -> (0, 0)
  line L4 (0, 0) -> (0, 13.945)
  constraints: 10 end point
revolve "Revolution2" cut sketch "_____18" angle 360 about axis through (5.5, 0, 0) along (0, -1, 0)
thread "Thread1" size "M4x0.7" class "6H" standard "ISO Metric profile" length 8.945
sketch "_____19" plane through (5.5, 0, 0) normal (1, 0, 0) x (0, 0, -1)
  line L0 (0, 0) -> (12.0767, -6.9725)
  line L1 (12.0767, -6.9725) -> (11.2662, -8.3763)
  line L2 (11.2662, -8.3763) -> (-0.8105, -1.4038)
  line L3 (-0.8105, -1.4038) -> (0, 0)
  line L4 (0, 0) -> (12.0767, -6.9725)
  constraints: 10 end point
revolve "Revolution3" cut sketch "_____19" angle 360 about axis through (5.5, 0, 0) along (0, 0.5, 0.8660254)
thread "Thread2" size "M4x0.7" class "6H" standard "ISO Metric profile" length 8.945 offset 0.1755
ref_plane "to_belt_XY" through (5.5, 0, 0) normal (-1, 0, 0) x (0, 0, -1)
ref_plane "to_belt_YZ" through (5.5, 0, 0) normal (0, 0, -1) x (0, -1, 0)
ref_plane "to_belt_ZX" through (5.5, 0, 0) normal (0, -1, 0) x (-1, 0, 0)
ref_plane "to_screw1_XY" through (5.5, 6.4, 0) normal (0, 1, 0) x (1, 0, 0)
ref_plane "to_screw1_YZ" through (5.5, 6.4, 0) normal (1, 0, 0) x (0, 0, -1)
ref_plane "to_screw1_ZX" through (5.5, 6.4, 0) normal (0, 0, -1) x (0, 1, 0)
ref_plane "to_screw2_XY" through (5.5, -2.5, -4.3301) normal (0, -0.5, -0.8660254) x (1, 0, 0)
ref_plane "to_screw2_YZ" through (5.5, -2.5, -4.3301) normal (1, 0, 0) x (0, -0.8660254, 0.5)
ref_plane "to_screw2_ZX" through (5.5, -2.5, -4.3301) normal (0, -0.8660254, 0.5) x (0, -0.5, -0.8660254)
body "Solid1"
